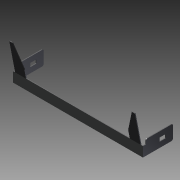
# Autodesk Inventor part: UB16NKG015F-NR
Saved by Autodesk Inventor 2015 SP1 (Build 190203100, 203)
## iProperties
Category: Electrical
Company: Autodesk Inc.
Created: 2014-12-16
Part Number: UB16NKG015F-NR
Catalog Web Link: http://www.nkkswitches.com/
Description: UB_ill_metal-Illuminated Pushbuttons - Series UB, metal
Vendor: NKK Switches
Document SubType Name: Modeling
Designer: Autodesk Inc.
Manufacturer: NKKSWITCHES
Mass: 0.0092607 g
Surface Area: 1.58359 cm^2
Volume: 0.0092607 cm^3
Density: 1 g/cm^3
Material: Generic
Appearance: PSOLRGB-234-234-234
PSOL_IDENT_2: RSION=},{LINEID=10},{LINESUBID=-1},{WBVAR=MT}  {NB=UBNK-metal_},{LINA=UBNK-metal_},{KT=DUMMY},{SRS=U
PSOL_IDENT_3: B},{MT=NK}
SUPPLIER: NKKSWITCHES
Title: UBNK-metal_
Author: Autodesk Inc.
Comments: Illuminated Pushbuttons - Series UB, metal
Autodesk Inventor part; units mm, degrees
sketch "Sketch_7" plane through (0, 0, 7.8994) normal (0, 0, 1) x (1, 0, 0)
  line L0 (-10.8712, 1.3208) -> (10.8712, 1.3208)
  line L1 (10.8712, 1.3208) -> (10.8712, 2.9972)
  line L2 (10.8712, 2.9972) -> (-10.8712, 2.9972)
  line L3 (-10.8712, 2.9972) -> (-10.8712, 1.3208)
  constraints: 8 end point
extrude "Extrusion1" add sketch "Sketch_7" against normal blind 0.127
sketch "Sketch_11" plane through (-10.9982, 0, 0) normal (1, 0, 0) x (0, 0, -1)
  line L0 (-7.8994, 1.3208) -> (-3.0734, 1.3208)
  arc A0 (-3.0734, 1.3208) -> (-2.8194, 1.5748) centre (-3.0734, 1.5748) ccw
  line L1 (-2.8194, 1.5748) -> (-2.8194, 3.5052)
  arc A1 (-2.8194, 3.5052) -> (-3.0734, 3.7592) centre (-3.0734, 3.5052) ccw
  line L2 (-3.0734, 3.7592) -> (-7.1374, 3.7592)
  arc A2 (-7.1374, 3.7592) -> (-7.3914, 3.5052) centre (-7.1374, 3.5052) ccw
  line L3 (-7.3914, 3.5052) -> (-7.3914, 2.9972)
  line L4 (-7.3914, 2.9972) -> (-7.8994, 2.9972)
  line L5 (-7.8994, 2.9972) -> (-7.8994, 1.3208)
  line L6 (-5.0546, 2.8448) -> (-5.0546, 2.2352)
  line L7 (-5.0546, 2.2352) -> (-4.0386, 2.2352)
  line L8 (-4.0386, 2.2352) -> (-4.0386, 2.8448)
  line L9 (-4.0386, 2.8448) -> (-5.0546, 2.8448)
  constraints: 20 end point, 6 point on circle, 3 centre point
extrude "Extrusion2" add sketch "Sketch_11" along normal blind 0.127
sketch "Sketch_13" plane through (10.9982, 0, 0) normal (1, 0, 0) x (0, 0, -1)
  line L0 (-7.8994, 1.3208) -> (-3.0734, 1.3208)
  arc A0 (-3.0734, 1.3208) -> (-2.8194, 1.5748) centre (-3.0734, 1.5748) ccw
  line L1 (-2.8194, 1.5748) -> (-2.8194, 3.5052)
  arc A1 (-2.8194, 3.5052) -> (-3.0734, 3.7592) centre (-3.0734, 3.5052) ccw
  line L2 (-3.0734, 3.7592) -> (-7.1374, 3.7592)
  arc A2 (-7.1374, 3.7592) -> (-7.3914, 3.5052) centre (-7.1374, 3.5052) ccw
  line L3 (-7.3914, 3.5052) -> (-7.3914, 2.9972)
  line L4 (-7.3914, 2.9972) -> (-7.8994, 2.9972)
  line L5 (-7.8994, 2.9972) -> (-7.8994, 1.3208)
  line L6 (-5.0546, 2.8448) -> (-5.0546, 2.2352)
  line L7 (-5.0546, 2.2352) -> (-4.0386, 2.2352)
  line L8 (-4.0386, 2.2352) -> (-4.0386, 2.8448)
  line L9 (-4.0386, 2.8448) -> (-5.0546, 2.8448)
  constraints: 20 end point, 6 point on circle, 3 centre point
extrude "Extrusion3" add sketch "Sketch_13" against normal blind 0.127
sketch "Sketch_17" plane through (0, 0, 0) normal (1, 0, 0) x (0, 1, 0)
  line L0 (8.128, 8.9027) -> (2.9972, 7.8994)
  line L1 (2.9972, 7.8994) -> (2.9972, 7.7726)
  line L2 (2.9972, 7.7726) -> (8.1519, 8.7806)
  line L3 (8.1519, 8.7806) -> (8.128, 8.9027)
  constraints: 8 end point
extrude "Extrusion4" add sketch "Sketch_17" along normal mid plane 21.336
sketch "Sketch_18" plane through (0, 0, 7.6454) normal (0, 0, 1) x (1, 0, 0)
  line L0 (-11.1252, 8.4328) -> (-11.1252, 2.9972)
  line L1 (-11.1252, 2.9972) -> (-10.6172, 2.9972)
  line L2 (-10.6172, 2.9972) -> (-10.6172, 8.0772)
  line L3 (-10.6172, 8.0772) -> (-10.1092, 8.0772)
  line L4 (-10.1092, 8.0772) -> (-8.78, 4.4254)
  line L5 (-8.78, 4.4254) -> (-8.78, 2.9972)
  line L6 (-8.78, 2.9972) -> (8.78, 2.9972)
  line L7 (8.78, 2.9972) -> (8.78, 4.4254)
  line L8 (8.78, 4.4254) -> (10.1092, 8.0772)
  line L9 (10.1092, 8.0772) -> (10.6172, 8.0772)
  line L10 (10.6172, 8.0772) -> (10.6172, 2.9972)
  line L11 (10.6172, 2.9972) -> (11.1252, 2.9972)
  line L12 (11.1252, 2.9972) -> (11.1252, 8.4328)
  line L13 (11.1252, 8.4328) -> (-11.1252, 8.4328)
  constraints: 28 end point
extrude "Extrusion5" cut sketch "Sketch_18" along normal blind 2.794
ref_plane "metal_XY" through (0, 0, 0) normal (0, 1, 0) x (1, 0, 0)
ref_plane "metal_YZ" through (0, 0, 0) normal (1, 0, 0) x (0, 0, -1)
ref_plane "metal_ZX" through (0, 0, 0) normal (0, 0, -1) x (0, 1, 0)
body "Solid1"
